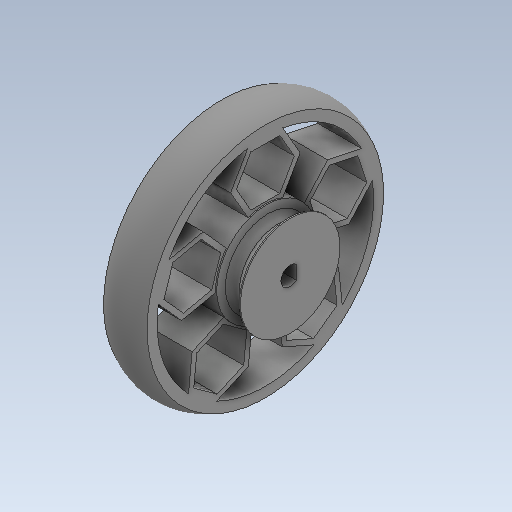
# Autodesk Inventor part: PulleyedWheelV1
Saved by Autodesk Inventor 2020 (Build 240168000, 168)
## iProperties
Created: 2023-12-21
Part Number: PulleyedWheelV1
Material: H TPU
Document SubType Name: Modeling
Designer: smz3rm
Density: 0.941117 g/cm^3
Appearance: Generic(1)
Mass: 7.67188 g
Surface Area: 75.5159 cm^2
Volume: 8.15189 cm^3
d0: 3.000 mm
d1: 1.000 mm
d3: 38.000 mm
d4: 3.000 mm
d6: 16.000 mm
d7: 4.000 mm
d8: 0.00 deg
d9: 38.000 mm
d10: 1.600 mm
d11: 0.800 mm
d16: 7.000 mm
d17: 0.00 deg
d20: 2.000 mm
d24: 1.000 mm
d26: 45.00 deg
Roundedness: 1.000 mm
BaseThickness: 3.000 mm
TopThickness: 1.778 mm
SideThickness: 4.000 mm
BodyWidth: 130.000 mm
BodyLength: 150.000 mm
BodyHeight: 30.000 mm
DriveMotorHeight: 15.000 mm
WheelDia: 40.000 mm
WheelWidth: 7.000 mm
WheelGrooveWidth: 4.000 mm
WheelGrooveDia: 16.000 mm
WheelSlotWidth: 20.000 mm
WheelPulleyDia: 2.000 mm
WheeGuardlSlotWidth: 14.000 mm
Author: smz3rm
Autodesk Inventor part; units mm, degrees
ref_plane "YZ Plane" through (0, 0, 0) normal (1, 0, 0) x (0, 1, 0)
ref_plane "XZ Plane" through (0, 0, 0) normal (0, 1, 0) x (-1, 0, 0)
ref_plane "XY Plane" through (0, 0, 0) normal (0, 0, 1) x (1, 0, 0)
sketch "Sketch1" plane through (0, 0, 0) normal (1, 0, 0) x (0, 1, 0)
  circle A0 centre (0, 0) radius 1.5
  line L0 (-26.6, 0) -> (26.6, 0) projected
  line L1 (1.118, -1) -> (-1.118, -1)
  circle A1 centre (0, 0) radius 8
  circle A2 centre (0, 0) radius 19
  circle A3 centre (0, 0) radius 16
  dimension "d0" = 3
  dimension "d1" = 1
  dimension "d3" = 38
  dimension "d4" = 3
  dimension "d6" = 16
  constraints: 4 centre point, 4 coincident, 2 end point, 2 point on circle, 1 horizontal
  measures "d0" diameter of A0
  measures "d1" distance between parallel lines of L0 L1
  measures "d3" diameter of A2
  measures "d4" radial gap between concentric circles of A2 A3
  measures "d6" diameter of A1
extrude "Extrusion1" add sketch "Sketch1" along normal blind 4 contours L1 A0 | A0 L0 A1 | L0 A1 A0
sketch "Sketch3" plane through (0, 0, 0) normal (0, 0, 1) x (1, 0, 0)
  line L0 (0, 8) -> (4, 8) projected
  line L1 (-0.8, 0) -> (4.8, 0) projected
  circle A0 centre (1.3858, 7) radius 1
  line L2 (0.4001, 6.8312) -> (0.2, 8)
  line L3 (0, 8) -> (4, 8) projected
  line L4 (0, 10) -> (4, 10) projected
  line L5 (0, 8) -> (4, 8) projected
  line L6 (3.8, 8) -> (2.0929, 6.2929)
  line L7 (3.8, 8) -> (3.8, 8)
  line L8 (3.8, 8) -> (4, 8)
  line L9 (4, -8) -> (4, 8) projected
  line L10 (4, 8) -> (4, 8)
  line L11 (0, -8) -> (0, 8) projected
  line L12 (0.2, 8) -> (0, 8)
  point P0 (0, 0)
  point P1 (1.3858, 8)
  point P2 (3.8, 8)
  dimension "d20" = 2
  dimension "d26" = 45
  dimension "d28" = 0.2
  constraints: 12 end point, 3 perpendicular, 3 tangent, 2 collinear, 2 point on circle, 2 point on line, 1 centre point, 1 vertical, 3 other
  measures "d20" diameter of A0
  measures "d26" angle of L0 L6
  measures "d28" distance of L0.end L6.start
revolve "Revolution1" cut sketch "Sketch3" angle 360 about axis through (-10, 0, 0) along (-1, 0, 0) contours L0 A0 L2 | L0 L6 A0 | A0
sketch "Sketch2" plane through (0, 0, 0) normal (-1, 0, 0) x (0, 0, 1)
  circle A0 centre (0, 0) radius 19
  circle A1 centre (0, 0) radius 17.4
  circle A2 centre (0, 0) radius 8 projected
  line L0 (-1, 1.118) -> (-1, -1.118) projected
  arc A3 (-1, -1.118) -> (-1, 1.118) centre (0, 0) ccw projected
  line L1 (2.7938, 17.1742) -> (5.5876, 12.3353)
  line L2 (5.5876, 12.3353) -> (2.7938, 7.4963)
  line L3 (2.7938, 7.4963) -> (-2.7938, 7.4963)
  line L4 (-2.7938, 7.4963) -> (-5.5876, 12.3353)
  line L5 (-5.5876, 12.3353) -> (-2.7938, 17.1742)
  line L6 (-2.7938, 17.1742) -> (2.7938, 17.1742)
  line L7 (0, -26.6) -> (0, 26.6) projected
  line L8 (-2.3319, 16.3742) -> (-4.6638, 12.3353)
  line L9 (-4.6638, 12.3353) -> (-2.3319, 8.2963)
  line L10 (-2.3319, 8.2963) -> (2.3319, 8.2963)
  line L11 (2.3319, 8.2963) -> (4.6638, 12.3353)
  line L12 (4.6638, 12.3353) -> (2.3319, 16.3742)
  line L13 (2.3319, 16.3742) -> (-2.3319, 16.3742)
  line L14 (-15.4704, 7.9642) -> (-10.0049, 9.1259)
  line L15 (-17.197, 2.6501) -> (-15.4704, 7.9642)
  line L16 (-13.4582, -1.5023) -> (-17.197, 2.6501)
  line L17 (-7.9927, -0.3406) -> (-13.4582, -1.5023)
  line L18 (-13.1727, -0.6237) -> (-8.6109, 0.3459)
  line L19 (-8.6109, 0.3459) -> (-7.1697, 4.7815)
  line L20 (-7.1697, 4.7815) -> (-10.2904, 8.2473)
  line L21 (-10.0049, 9.1259) -> (-6.2661, 4.9735)
  line L22 (-6.2661, 4.9735) -> (-7.9927, -0.3406)
  line L23 (-10.2904, 8.2473) -> (-14.8522, 7.2777)
  line L24 (-14.8522, 7.2777) -> (-16.2934, 2.8422)
  line L25 (-16.2934, 2.8422) -> (-13.1727, -0.6237)
  line L26 (-12.355, -12.2521) -> (-11.7709, -6.6952)
  line L27 (-7.8346, -15.5364) -> (-12.355, -12.2521)
  line L28 (-2.7301, -13.2637) -> (-7.8346, -15.5364)
  line L29 (-2.146, -7.7068) -> (-2.7301, -13.2637)
  line L30 (-3.4774, -12.7208) -> (-2.9899, -8.0825)
  line L31 (-2.9899, -8.0825) -> (-6.763, -5.3412)
  line L32 (-6.763, -5.3412) -> (-11.0236, -7.2381)
  line L33 (-11.7709, -6.6952) -> (-6.6664, -4.4225)
  line L34 (-6.6664, -4.4225) -> (-2.146, -7.7068)
  line L35 (-11.0236, -7.2381) -> (-11.5111, -11.8764)
  line L36 (-11.5111, -11.8764) -> (-7.738, -14.6177)
  line L37 (-7.738, -14.6177) -> (-3.4774, -12.7208)
  line L38 (7.8346, -15.5364) -> (2.7301, -13.2637)
  line L39 (12.355, -12.2521) -> (7.8346, -15.5364)
  line L40 (11.7709, -6.6952) -> (12.355, -12.2521)
  line L41 (6.6664, -4.4225) -> (11.7709, -6.6952)
  line L42 (11.0236, -7.2381) -> (6.763, -5.3412)
  line L43 (6.763, -5.3412) -> (2.9899, -8.0825)
  line L44 (2.9899, -8.0825) -> (3.4774, -12.7208)
  line L45 (2.7301, -13.2637) -> (2.146, -7.7068)
  line L46 (2.146, -7.7068) -> (6.6664, -4.4225)
  line L47 (3.4774, -12.7208) -> (7.738, -14.6177)
  line L48 (7.738, -14.6177) -> (11.5111, -11.8764)
  line L49 (11.5111, -11.8764) -> (11.0236, -7.2381)
  line L50 (17.197, 2.6501) -> (13.4582, -1.5023)
  line L51 (15.4704, 7.9642) -> (17.197, 2.6501)
  line L52 (10.0049, 9.1259) -> (15.4704, 7.9642)
  line L53 (6.2661, 4.9735) -> (10.0049, 9.1259)
  line L54 (10.2904, 8.2473) -> (7.1697, 4.7815)
  line L55 (7.1697, 4.7815) -> (8.6109, 0.3459)
  line L56 (8.6109, 0.3459) -> (13.1727, -0.6237)
  line L57 (13.4582, -1.5023) -> (7.9927, -0.3406)
  line L58 (7.9927, -0.3406) -> (6.2661, 4.9735)
  line L59 (13.1727, -0.6237) -> (16.2934, 2.8422)
  line L60 (16.2934, 2.8422) -> (14.8522, 7.2777)
  line L61 (14.8522, 7.2777) -> (10.2904, 8.2473)
  point P0 (0, 12.3353)
  point P1 (2.7938, 7.4963)
  point P2 (-15.4704, 7.9642)
  point P3 (-6.2661, 4.9735)
  point P4 (-17.197, 2.6501)
  point P5 (-7.9927, -0.3406)
  point P6 (-6.6664, -4.4225)
  point P7 (-12.355, -12.2521)
  point P8 (-7.8346, -15.5364)
  point P9 (-2.146, -7.7068)
  point P10 (7.8346, -15.5364)
  point P11 (12.355, -12.2521)
  point P12 (6.6664, -4.4225)
  point P13 (7.9927, -0.3406)
  point P14 (17.197, 2.6501)
  point P15 (15.4704, 7.9642)
  point P16 (6.2661, 4.9735)
  dimension "d9" = 38
  dimension "d10" = 1.6
  dimension "d11" = 0.8
  dimension "d31" = 360
  constraints: 120 end point, 2 centre point, 2 coincident, 2 point on circle, 1 point on line, 141 other
  measures "d9" diameter of A0
  measures "d10" radial gap between concentric circles of A0 A1
  measures "d11" distance between parallel lines of L5 L8
extrude "Extrusion2" add sketch "Sketch2" along normal blind 7 contours A0 L7 A1 | L7 A1 A0 | L7 L6 A1 | A1 L6 L7 | L1 L2 A2 L7 L10 L11 L12 L13 L6 | L6 L7 L13 L8 L9 L10 A2 L4 L5 | A1 L27 | L27 L26 L33 A2 L29 L28 | L39 A1 | L38 L45 A2 L41 L40 L39 | L7 A3 L3 A2 L58 L46 | A2 L34 L22 L3 L7 A3 L0 | A1 L51 | L51 L50 L57 A2 L53 L52 | L15 A1 | L14 L21 A2 L17 L16 L15 | A2 L34 | L46 A2 | L3 L7 A2 | A2 L7 L3 | A2 L58 | L22 A2
sketch "Sketch4" plane through (0, 0, 0) normal (0, 0, 1) x (1, 0, 0)
  line L0 (0, 19) -> (-7, 19) projected
  line L1 (-7, 19) -> (-7, -19) projected
  arc A0 (0, 19) -> (-7, 19) centre (-3.5, 13.375) ccw
  line L2 (-15.6, 0) -> (2.6, 0) projected
  point P0 (0, 0)
  point P1 (-3.5, 20)
  dimension "d24" = 1
  constraints: 3 point on circle, 1 centre point
  measures "d24" distance from line of L0 point (-3.5, 20)
revolve "Revolution2" add sketch "Sketch4" angle 360 about axis through (-10, 0, 0) along (1, 0, 0)
equation "\"d6\" = WheelGrooveDia"
equation "\"d7\" = WheelGrooveWidth"
equation "\"d20\" = WheelPulleyDia"
equation "\"d9\" = WheelDia - 2 * Roundedness"
equation "\"d16\" = WheelWidth"
equation "\"d24\" = Roundedness"
equation "\"Roundedness\" = 1"
equation "\"WheelGrooveDia\" = 16"
equation "\"WheelGrooveWidth\" = 4"
equation "\"WheelPulleyDia\" = 2"
equation "\"WheelDia\" = 40"
equation "\"WheelWidth\" = 7"
body "Solid1"
